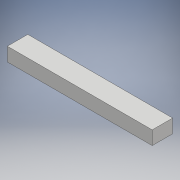
# Autodesk Inventor part: Cadru_1
Saved by Autodesk Inventor 2017 (Build 210142000, 142)
## iProperties
Created: 2017-06-13
Part Number: Cadru_1
Material: Generic
Document SubType Name: Modeling
Designer: crush
Density: 1 g/cm^3
Appearance: Default
Author: crush
Autodesk Inventor part; units mm, degrees
ref_plane "YZ Plane" through (0, 0, 0) normal (1, 0, 0) x (0, 1, 0)
ref_plane "XZ Plane" through (0, 0, 0) normal (0, 1, 0) x (-1, 0, 0)
ref_plane "XY Plane" through (0, 0, 0) normal (0, 0, 1) x (1, 0, 0)
sketch "Sketch1" plane through (0, 0, 0) normal (0, 1, 0) x (-1, 0, 0)
  line L0 (0, 0) -> (-425, 0)
  line L1 (-425, 0) -> (-425, -40)
  line L2 (-425, -40) -> (0, -40)
  line L3 (0, -40) -> (0, 0)
  dimension "d0" = 425
  dimension "d1" = 40
  constraints: 8 end point, 2 parallel, 1 horizontal, 1 perpendicular
  measures "d0" distance of L1.end L2.end
  measures "d1" distance of L2.end L0.start
extrude "Extrusion1" add sketch "Sketch1" along normal blind 60
body "Solid1"
